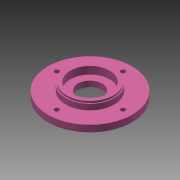
# Autodesk Inventor part: 装填盘轴盖
Saved by Autodesk Inventor 2015 (Build 190159000, 159)
## iProperties
Created: 2017-05-18
Part Number: 装填盘轴盖
Material: 常规
Document SubType Name: Modeling
Designer: Administrator
Density: 1 g/cm^3
Appearance: 粉红色
Author: Administrator
Autodesk Inventor part; units mm, degrees
ref_plane "YZ Plane" through (0, 0, 0) normal (1, 0, 0) x (0, 1, 0)
ref_plane "XZ Plane" through (0, 0, 0) normal (0, 1, 0) x (-1, 0, 0)
ref_plane "XY Plane" through (0, 0, 0) normal (0, 0, 1) x (1, 0, 0)
sketch "草图1" plane through (0, 0, 0) normal (0, 0, 1) x (1, 0, 0)
  circle A0 centre (0, 0) radius 45
  dimension "d0" = 90
  constraints: 1 centre point, 1 coincident
  measures "d0" diameter of A0
extrude "拉伸1" add sketch "草图1" along normal blind 7
sketch "草图2" plane through (0, 0, 7) normal (0, 0, 1) x (1, 0, 0)
  circle A0 centre (0, 0) radius 26
  circle A1 centre (0, 0) radius 21
  dimension "d3" = 52
  dimension "d4" = 42
  constraints: 2 centre point, 2 coincident
  measures "d3" diameter of A0
  measures "d4" diameter of A1
extrude "拉伸2" add sketch "草图2" along normal blind 8
sketch "草图3" plane through (0, 0, 15) normal (0, 0, 1) x (1, 0, 0)
  circle A0 centre (0, 0) radius 26
  circle A1 centre (0, 0) radius 25
  dimension "d7" = 52
  dimension "d8" = 50
  constraints: 2 centre point, 2 coincident
  measures "d7" diameter of A0
  measures "d8" diameter of A1
extrude "拉伸3" cut sketch "草图3" against normal blind 2
sketch "草图4" plane through (0, 0, 7) normal (0, 0, 1) x (1, 0, 0)
  circle A0 centre (0, 0) radius 13
  dimension "d11" = 26
  constraints: 1 centre point, 1 coincident
  measures "d11" diameter of A0
extrude "拉伸4" cut sketch "草图4" against normal through all
sketch "草图5" plane through (0, 0, 0) normal (0, 0, -1) x (-1, 0, 0)
  circle A0 centre (0, -35.5) radius 2.5
  circle A1 centre (35.5, 0) radius 2.5
  circle A2 centre (-35.5, 0) radius 2.5
  circle A3 centre (0, 35.5) radius 2.5
  line L0 (0, 0) -> (-3.8614, 0)
  line L1 (0, 0) -> (0, -7.2667)
  dimension "d15" = 5
  dimension "d16" = 5
  dimension "d17" = 5
  dimension "d18" = 5
  dimension "d19" = 35.5
  dimension "d20" = 35.5
  dimension "d21" = 35.5
  dimension "d22" = 35.5
  dimension "d23" = 7.2667
  dimension "d24" = 3.8614
  constraints: 4 centre point, 4 end point, 4 point on line, 1 horizontal, 1 vertical
  measures "d15" diameter of A0
  measures "d16" diameter of A1
  measures "d17" diameter of A2
  measures "d18" diameter of A3
  measures "d19" distance of L0.start A0.centre
  measures "d20" distance of A2.centre L0.start
  measures "d21" distance of L0.start A1.centre
  measures "d22" distance of L0.start A3.centre
  measures "d23" distance of L0.start L1.end
  measures "d24" distance of L0.start L0.end
extrude "拉伸5" cut sketch "草图5" against normal through all
sketch "草图6" plane through (0, 0, 0) normal (0, 0, -1) x (-1, 0, 0)
  circle A0 centre (0, 0) radius 22.5
  dimension "d27" = 45
  constraints: 1 centre point, 1 coincident
  measures "d27" diameter of A0
extrude "拉伸6" cut sketch "草图6" against normal blind 1
fillet "圆角1" radius 0.5 2 edges at (22.5, 0, 0) (22.5, 0, 1)
equation "\"d12\" = d11"
